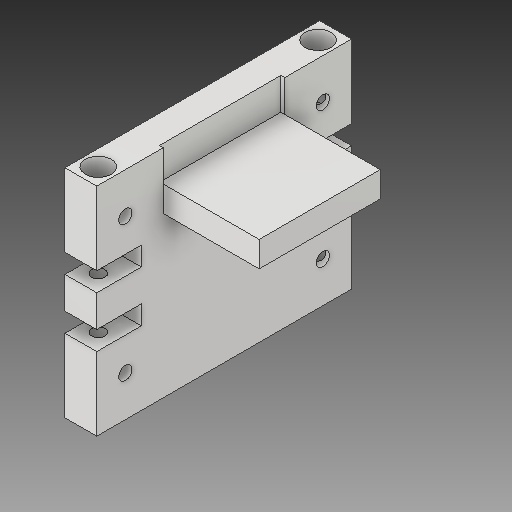
# Autodesk Inventor part: КВ33.044.604 - Щека 2 каретка оси Y
Saved by Autodesk Inventor 2019 (Build 230136000, 136)
## iProperties
Created: 2019-08-12
Part Number: КВ33.044.604 - Щека 2 каретка оси Y
Material: Пластик АБС
Document SubType Name: Modeling
Designer: Петров Иван
Density: 1.06 g/cm^3
Appearance: Гладкий — белый
Author: Петров Иван
Autodesk Inventor part; units mm, degrees
ref_plane "YZ Plane" through (0, 0, 0) normal (1, 0, 0) x (0, 1, 0)
ref_plane "XZ Plane" through (0, 0, 0) normal (0, 1, 0) x (-1, 0, 0)
ref_plane "XY Plane" through (0, 0, 0) normal (0, 0, 1) x (1, 0, 0)
sketch "Эскиз1" plane through (0, 0, 0) normal (1, 0, 0) x (0, 1, 0)
  circle A0 centre (20, 15) radius 1.5
  circle A1 centre (-20, -15) radius 1.5
  circle A2 centre (-20, 15) radius 1.5
  circle A3 centre (20, -15) radius 1.5
  circle A4 centre (-21.3, -31) radius 2.1
  circle A5 centre (21.3, -31) radius 2.1
  circle A6 centre (-21.3, 31) radius 2.1
  circle A7 centre (21.3, 31) radius 2.1
  line L0 (-11, -40) -> (-11, -26)
  line L1 (-11, -26) -> (-5, -26)
  line L2 (-5, -26) -> (-5, -40)
  line L3 (-5, -40) -> (5, -40)
  line L4 (5, -40) -> (5, -26)
  line L5 (5, -26) -> (11, -26)
  line L6 (11, -26) -> (11, -40)
  line L7 (11, -40) -> (34, -40)
  line L8 (34, -40) -> (34, 40)
  line L9 (34, 40) -> (11, 40)
  line L10 (11, 40) -> (11, 26)
  line L11 (11, 26) -> (5, 26)
  line L12 (5, 26) -> (5, 40)
  line L13 (5, 40) -> (-5, 40)
  line L14 (-5, 40) -> (-5, 26)
  line L15 (-5, 26) -> (-11, 26)
  line L16 (-11, 26) -> (-11, 40)
  line L17 (-11, 40) -> (-34, 40)
  line L18 (-34, 40) -> (-34, -40)
  line L19 (-34, -40) -> (-11, -40)
  point P0 (0, 0)
  constraints: 40 end point, 8 centre point
extrude "Выдавливание1" add sketch "Эскиз1" along normal blind 10 contours A0 | A1 | A2 | A3 | L19 L18 L17 L16 L15 L14 L13 L12 L11 L10 L9 L8 L7 L6 L5 L4 L3 L2 L1 L0
sketch "Эскиз2" plane through (10, 0, 0) normal (1, 0, 0) x (0, 0, -1)
  circle A0 centre (15, -20) radius 1.5
  circle A1 centre (-15, 20) radius 1.5
  circle A2 centre (15, 20) radius 1.5
  circle A3 centre (-15, -20) radius 1.5
  circle A4 centre (-31, 21.48) radius 2.1
  circle A5 centre (-31, -21.48) radius 2.1
  circle A6 centre (31, 21.48) radius 2.1
  circle A7 centre (31, -21.48) radius 2.1
  line L0 (-40, 11) -> (-26, 11)
  line L1 (-26, 11) -> (-26, 5)
  line L2 (-26, 5) -> (-40, 5)
  line L3 (-40, 5) -> (-40, -5)
  line L4 (-40, -5) -> (-26, -5)
  line L5 (-26, -5) -> (-26, -11)
  line L6 (-26, -11) -> (-40, -11)
  line L7 (-40, -11) -> (-40, -34)
  line L8 (-40, -34) -> (40, -34)
  line L9 (40, -34) -> (40, -11)
  line L10 (40, -11) -> (26, -11)
  line L11 (26, -11) -> (26, -5)
  line L12 (26, -5) -> (40, -5)
  line L13 (40, -5) -> (40, 5)
  line L14 (40, 5) -> (26, 5)
  line L15 (26, 5) -> (26, 11)
  line L16 (26, 11) -> (40, 11)
  line L17 (40, 11) -> (40, 34)
  line L18 (40, 34) -> (-40, 34)
  line L19 (-40, 34) -> (-40, 11)
  line L20 (-15, 20) -> (-15, 24)
  line L21 (-15, 20) -> (-19, 20)
  line L22 (-19, 20) -> (-19, 24)
  line L23 (15, 20) -> (19, 20)
  line L24 (19, 20) -> (19, 16)
  line L25 (-19, 24) -> (19, 24)
  line L26 (19, 24) -> (19, 16)
  line L27 (19, 16) -> (-19, 16)
  line L28 (-19, 16) -> (-19, 24)
  point P0 (0, 0)
  point P1 (0, 0)
  dimension "d4" = 4
  dimension "d5" = 4
  dimension "d6" = 4
  dimension "d7" = 4
  constraints: 58 end point, 8 centre point, 3 horizontal, 3 perpendicular, 2 parallel, 1 vertical
  measures "d4" distance of L20.start L20.end
  measures "d5" distance of L20.start L21.end
  measures "d6" distance of L23.start L23.end
  measures "d7" distance of L23.end L24.end
extrude "Выдавливание2" add sketch "Эскиз2" along normal blind 30 contours A1 L21 L20 | A2 | A1 L20 L25 L26 L24 L27 L28 L21 | L20 L21 A1 | A1 L21 L22 L25 L20
sketch "Эскиз3" plane through (0, 34, 40) normal (0, 1, 0) x (1, 0, 0)
  line L0 (0, 0) -> (10, 0) projected
  line L1 (5, 0) -> (5, 5.5)
  line L2 (0, 80) -> (10, 80) projected
  line L3 (5, 80) -> (5, 74.5)
  circle A0 centre (5, 5.5) radius 2.1
  circle A1 centre (5, 74.5) radius 2.1
  point P0 (0, 40)
  dimension "d11" = 5.5
  dimension "d12" = 5.5
  dimension "d13" = 4.2
  dimension "d14" = 4.2
  constraints: 4 end point, 2 centre point, 2 coincident, 2 midpoint, 2 vertical
  measures "d11" distance of L1.start L1.end
  measures "d12" distance of L3.start L3.end
  measures "d13" diameter of A0
  measures "d14" diameter of A1
extrude "Выдавливание3" cut sketch "Эскиз3" against normal through all
sketch "Эскиз4" plane through (0, 34, 40) normal (0, 1, 0) x (1, 0, 0)
  circle A0 centre (5, 5.5) radius 2.1 projected
  circle A1 centre (5, 5.5) radius 4.1
  circle A2 centre (5, 74.5) radius 2.1 projected
  circle A3 centre (5, 74.5) radius 4.1
  point P0 (0, 40)
  dimension "d17" = 8.2
  dimension "d18" = 8.2
  constraints: 2 centre point, 2 coincident
  measures "d17" diameter of A1
  measures "d18" diameter of A3
extrude "Выдавливание4" cut sketch "Эскиз4" against normal blind 20 contours A0 | A1 | A2 | A3
sketch "Эскиз5" plane through (0, -34, -40) normal (0, -1, 0) x (1, 0, 0)
  circle A0 centre (5, 74.5) radius 2.1 projected
  circle A1 centre (5, 74.5) radius 4.1
  circle A2 centre (5, 5.5) radius 2.1 projected
  circle A3 centre (5, 5.5) radius 4.1
  point P0 (0, 40)
  dimension "d21" = 8.2
  dimension "d22" = 8.2
  constraints: 2 centre point, 2 coincident
  measures "d21" diameter of A1
  measures "d22" diameter of A3
extrude "Выдавливание5" cut sketch "Эскиз5" against normal blind 20 contours A0 | A1 | A2 | A3
sketch "Эскиз8" plane through (0, 34, 40) normal (0, 1, 0) x (1, 0, 0)
  line L0 (10, 0) -> (10, 80) projected
  line L1 (10, 20.8795) -> (8.8, 20.8795)
  line L2 (8.8, 20.8795) -> (8.8, 59)
  line L3 (8.8, 59) -> (10, 59)
  line L4 (10, 59) -> (10, 20.8795)
  point P0 (0, 40)
  dimension "d34" = 1.2
  constraints: 8 end point, 2 parallel, 1 horizontal, 1 perpendicular, 1 point on line
  measures "d34" distance of L2.end L3.end
extrude "Выдавливание8" cut sketch "Эскиз8" against normal blind 10
equation "\"d12\" = d11"
equation "\"d14\" = d13"
